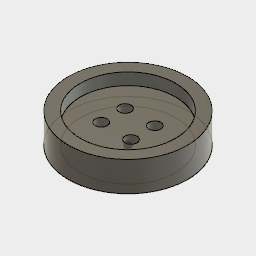
纽扣 (Autodesk Fusion 360 design; units mm, degrees)
Autodesk Fusion 360 part; units mm, degrees
sketch "草图1" plane through (0, 0, 0) normal (0, 1, 0) x (1, 0, 0)
  circle A0 centre (0, 0) radius 10
  circle A1 centre (0, 0) radius 8
  dimension "d1" = 20
  dimension "d2" = 2
  measures "d1" diameter of A0
surface "拉伸1" add extruded along (0, 1, 0) between 0 and 3 path "草图1" along A1 makes body 1
surface "拉伸2" add extruded along (0, 1, 0) between 0 and 5 path "草图1" along A0 separate body makes body 2
extrude "拉伸3" add sketch "草图1" along normal blind 3 separate body contours A1 makes body 3
extrude "拉伸4" add sketch "草图1" along normal blind 5 separate body makes body 4
cylinder "圆柱体基本要素1" add diameter 2 height 20 placed x (1, 0, 0) y (0, 0, -1) z (0, 1, 0) at (24, 0, 0) separate body makes body 5
move_body "移动1" bodies 5 to x (0.996224, 0.00033, 0.086824) y (0.00033, 0.999971, -0.007596) z (-0.086824, 0.007596, 0.996195) at (-23.6461, -5.1941, -1.9357)
pattern_linear "R-阵列1" count 2 spacing 4 along (0, 0, 1) count 2 spacing 5 along (1, 0, 0) of bodies 5 makes body 6 at (1.2503, 8.1479, 4.2324) makes body 7 at (6.2503, 8.1479, 0.2324) makes body 8 at (6.2503, 8.1479, 4.2324)
move_face "MoveFace1" to x (1, 0, 0) y (0, 1, 0) z (0, 0, 1) at (-2.8461, 0.803, -2.1794) 4 faces at (1.2503, 8.1479, 4.2324) (1.2503, 8.1479, 0.2324) (6.2503, 8.1479, 4.2324) (6.2503, 8.1479, 0.2324) on bodies 5 6 7 8
combine "合并1" operation cut target body 3 tool bodies 7 8 6 5
combine "合并2" operation add target body 4 tool bodies 3
